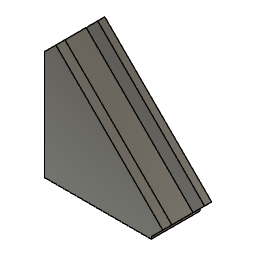
Elvf3 (Autodesk Fusion 360 design; units mm, degrees)
Autodesk Fusion 360 part; units mm, degrees
sketch "Sketch1" plane through (0, 0, 0) normal (1, 0, 0) x (0, 1, 0)
sketch "Sketch2" plane through (0, 0, 0) normal (0, 0, 1) x (1, 0, 0)
  line L0 (40, -30) -> (-40, -30)
  line L1 (-40, -30) -> (-40, 30)
  line L2 (-40, 30) -> (40, 30)
  line L3 (40, 30) -> (40, -30)
  constraint horizontal L0
  constraint vertical L1
  constraint horizontal L2
  constraint vertical L3
sketch "Sketch3" plane through (0, 0, 5) normal (0, 0, 1) x (-1, 0, 0)
  line L0 (-35, -25) -> (35, -25)
  line L1 (35, -25) -> (35, 25)
  line L2 (35, 25) -> (-35, 25)
  line L3 (-35, 25) -> (-35, -25)
  line L4 (57.1033, -33.9339) -> (188.0378, -33.9339)
  line L5 (188.0378, -33.9339) -> (188.0378, 25.9351)
  line L6 (188.0378, 25.9351) -> (57.1033, 25.9351)
  line L7 (57.1033, 25.9351) -> (57.1033, -33.9339)
  constraint horizontal L4
  constraint vertical L5
  constraint horizontal L6
  constraint vertical L7
extrude "Extrude2" add sketch "Sketch3" along normal blind 60 contours L4 L5 L6 L7
move_face "MoveFace1" to x (0.866025, 0, -0.5) y (0, 1, 0) z (0.5, 0, 0.866025) at (-45.0024, 0, -37.9511) 1 faces at (-144.3929, -5.9788, 65)
move_face "MoveFace2" to x (0.965926, 0, -0.258819) y (0, 1, 0) z (0.258819, 0, 0.965926) at (-29.2426, 0, -33.9791) 1 faces at (-144.3929, -5.9788, 94.4876)
sketch "Sketch4" plane through (-24.7999, 0, -24.7999) normal (0.707107, 0, 0.707107) x (0, 1, 0)
  line L0 (-25.9351, 45.6839) -> (33.9339, 45.6839)
  line L1 (33.9339, 45.6839) -> (33.9339, 230.8533)
  line L2 (33.9339, 230.8533) -> (-25.9351, 230.8533)
  line L3 (-25.9351, 230.8533) -> (-25.9351, 45.6839)
  line L4 (-14.831, 45.6839) -> (-14.831, 230.8533)
  line L5 (25.3011, 45.6839) -> (25.3011, 230.8533)
  constraint coincident L0 L4.start
  constraint coincident L2 L4.end
  constraint perpendicular L2 L4
  constraint coincident L0 L5.start
  constraint coincident L2 L5.end
  constraint perpendicular L2 L5
extrude "Extrude3" add sketch "Sketch4" along normal blind 20 contours L0 L2 L3 L4 | L0 L1 L2 L5
sketch "Sketch7" plane through (0, 0, 0) normal (0, 0, 1) x (1, 0, 0)
fillet "Fillet1" [suppressed]
fillet "Fillet2" [suppressed]
fillet "Fillet3" [suppressed]
sketch "Sketch5" plane through (0, 0, 0) normal (0, 1, 0) x (1, 0, 0)
sketch "Sketch6" plane through (0, 0, 0) normal (0, 0, 1) x (1, 0, 0)
